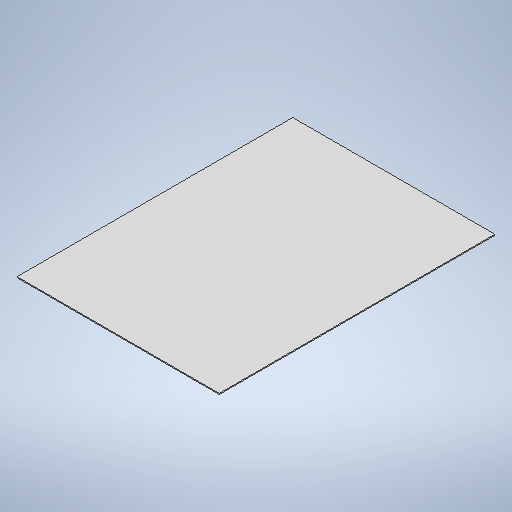
# Autodesk Inventor part: aile
Saved by Autodesk Inventor 2025.1 (Build 291241000, 241)
## iProperties
Created: 2025-07-16
Part Number: aile
Material: Générique
Document SubType Name: Modeling
Designer: chapuzet
Density: 1 g/cm^3
Appearance: Par défaut
Author: chapuzet
Autodesk Inventor part; units mm, degrees
ref_plane "YZ Plane" through (0, 0, 0) normal (1, 0, 0) x (0, 1, 0)
ref_plane "XZ Plane" through (0, 0, 0) normal (0, 1, 0) x (-1, 0, 0)
ref_plane "XY Plane" through (0, 0, 0) normal (0, 0, 1) x (1, 0, 0)
sketch "Esquisse1" plane through (0, 0, 0) normal (0, 1, 0) x (-1, 0, 0)
  line L0 (-110, 150) -> (110, 150)
  line L1 (110, 150) -> (110, -150)
  line L2 (110, -150) -> (-110, -150)
  line L3 (-110, -150) -> (-110, 150)
  line L4 (-110, 150) -> (110, -150) construction
  line L5 (110, 150) -> (-110, -150) construction
  point P0 (0, 0)
  dimension "d0" = 220
  dimension "d1" = 300
  constraints: 12 end point, 2 midpoint, 2 parallel, 1 horizontal, 1 perpendicular
  measures "d0" distance of L1.end L2.end
  measures "d1" distance of L0.end L1.end
extrude "Extrusion1" add sketch "Esquisse1" along normal blind 1
